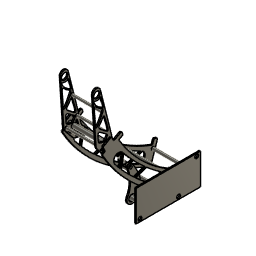
Klapptriebwerk v25 (Autodesk Fusion 360 design; units mm, degrees)
Autodesk Fusion 360 part; units mm, degrees
note: some values were not read from the file. Set by a fixed rule: which face or edge a step refers to.
(part 1 of 2)
sketch "Sketch2" plane through (0, 0, 0) normal (1, 0, 0) x (0, 1, 0)
  line L0 (125, -60) -> (-125, -60)
  line L1 (-125, -60) -> (-125, 60)
  line L2 (-125, 60) -> (125, 60)
  line L3 (125, 60) -> (125, -60)
  line L4 (125, -60) -> (-125, 60) construction
  line L5 (-125, -60) -> (125, 60) construction
  arc A0 (-186.1426, 249.5286) -> (95.8875, 14.6255) centre (286.6925, 530.468) ccw
  arc A1 (-250.577, 231.1913) -> (89.5042, -52.0625) centre (286.6925, 530.468) ccw
  line L6 (112.4731, 8.7903) -> (92.6771, -50.4864)
  line L7 (-240.9623, 242.2177) -> (-248.2082, 255.3516)
  line L8 (-247.2269, 258.7482) -> (-218.7703, 274.4476)
  line L9 (-215.3737, 273.4663) -> (-208.1278, 260.3325)
  line L10 (-223.3374, 249.0861) -> (-254.8183, 306.148) construction
  line L11 (-194.8808, 264.7856) -> (-204.7312, 259.3511)
  line L12 (-241.9437, 238.8211) -> (-249.6006, 234.5968)
  line L13 (-194.8808, 264.7856) -> (-179.3789, 273.3379)
  line L14 (-175.9823, 272.3566) -> (-171.1517, 263.6007)
  line L15 (-172.133, 260.2041) -> (-185.201, 252.9945)
  line L16 (112.4731, 8.7903) -> (118.0165, 25.3892)
  line L17 (116.4371, 28.5523) -> (106.9521, 31.72)
  line L18 (103.7889, 30.1406) -> (99.1261, 16.1784)
  arc A2 (-185.201, 252.9945) -> (-186.1426, 249.5286) centre (-183.9934, 250.8056) ccw
  arc A3 (-172.133, 260.2041) -> (-171.1517, 263.6007) centre (-173.3407, 262.3931) ccw
  arc A4 (-175.9823, 272.3566) -> (-179.3789, 273.3379) centre (-178.1713, 271.1489) ccw
  arc A5 (-208.1278, 260.3325) -> (-204.7312, 259.3511) centre (-205.9388, 261.5401) ccw
  arc A6 (-215.3737, 273.4663) -> (-218.7703, 274.4476) centre (-217.5627, 272.2586) ccw
  arc A7 (-247.2269, 258.7482) -> (-248.2082, 255.3516) centre (-246.0193, 256.5592) ccw
  arc A8 (-241.9437, 238.8211) -> (-240.9623, 242.2177) centre (-243.1513, 241.0101) ccw
  arc A9 (-249.6006, 234.5968) -> (-250.577, 231.1913) centre (-248.3929, 232.4079) ccw
  arc A10 (89.5042, -52.0625) -> (92.6771, -50.4864) centre (90.3058, -49.6945) ccw
  arc A11 (118.0165, 25.3892) -> (116.4371, 28.5523) centre (115.6452, 26.1811) ccw
  arc A12 (106.9521, 31.72) -> (103.7889, 30.1406) centre (106.1602, 29.3487) ccw
  arc A13 (95.8875, 14.6255) -> (99.1261, 16.1784) centre (96.7548, 16.9703) ccw
  arc A14 (8.8006, 55.8354) -> (95.8875, 14.6255) centre (286.6925, 530.468) ccw
  arc A15 (10.0637, 57.9928) -> (96.7548, 16.9703) centre (286.6925, 530.468) ccw
  line L19 (96.7548, 16.9703) -> (95.8875, 14.6255)
  line L20 (10.0637, 57.9928) -> (8.8006, 55.8354)
  arc A16 (-94.5095, 47.8604) -> (89.5042, -52.0625) centre (286.6925, 530.468) ccw
  arc A17 (-96.0591, 45.8986) -> (88.7027, -54.4305) centre (286.6925, 530.468) ccw
  line L21 (88.7027, -54.4305) -> (89.5042, -52.0625)
  line L22 (-96.0591, 45.8986) -> (-94.5095, 47.8604)
  line L23 (324.1005, 496.8726) -> (249.2844, 496.8726)
  line L24 (249.2844, 496.8726) -> (249.2844, 564.0634)
  line L25 (249.2844, 564.0634) -> (324.1005, 564.0634)
  line L26 (324.1005, 564.0634) -> (324.1005, 496.8726)
  line L27 (324.1005, 496.8726) -> (249.2844, 564.0634) construction
  line L28 (249.2844, 496.8726) -> (324.1005, 564.0634) construction
  circle A18 centre (-223.3374, 249.0861) radius 15
  circle A19 centre (-223.3374, 249.0861) radius 8.5
  point P0 (-249.4159, 257.5405)
  point P1 (-216.5813, 275.6552)
  point P2 (-206.9201, 258.1435)
  point P3 (-177.1899, 274.5456)
  point P4 (-169.944, 261.4117)
  point P5 (-187.4558, 251.7506)
  point P6 (118.8084, 27.7604)
  point P7 (104.5808, 32.5119)
  point P8 (286.6925, 530.468)
  point P9 (286.6925, 530.468)
  dimension "d1" = 250
  dimension "d2" = 120
  dimension "d12" = 20
  dimension "d13" = 400
  dimension "d14" = 550
  dimension "d17" = 37.5
  dimension "d18" = 13.75
  dimension "d19" = 20
  dimension "d20" = 15
  dimension "d22" = 15
  dimension "d23" = 20
  dimension "d24" = 2.5
  dimension "d25" = -2.5
  dimension "d26" = 2.5
  dimension "d44" = 30
  dimension "d45" = 17
  constraint horizontal L0
  constraint perpendicular L0 L1
  constraint parallel L0 L2
  constraint parallel L1 L3
  constraint coincident L4 origin
  constraint coincident L5 origin
  constraint perpendicular L7 L8
  constraint perpendicular L9 L11
  constraint perpendicular L10 L11
  constraint perpendicular L7 L11
  constraint symmetric L7 L9 L10
  constraint collinear L11 L12
  constraint coincident L10.start L11
  constraint parallel L11 L13
  constraint perpendicular L13 L14
  constraint coincident A0 P5
  constraint perpendicular L14 L15
  constraint parallel L6 L16
  constraint perpendicular L16 L17
  constraint perpendicular L17 L18
  constraint concentric A0 A1
  constraint tangent L15 A2
  constraint tangent A0 A2
  constraint coincident P4 L14
  constraint coincident P4 L15
  constraint tangent L14 A3
  constraint tangent L15 A3
  constraint equal A2 A3
  constraint coincident P3 L13
  constraint coincident P3 L14
  constraint tangent L13 A4
  constraint tangent L14 A4
  constraint equal A2 A4
  constraint coincident P2 L9
  constraint coincident P2 L11
  constraint tangent L9 A5
  constraint tangent L11 A5
  constraint equal A2 A5
  constraint coincident P1 L8
  constraint coincident P1 L9
  constraint tangent L8 A6
  constraint tangent L9 A6
  constraint equal A2 A6
  constraint coincident P0 L7
  constraint coincident P0 L8
  constraint tangent L7 A7
  constraint tangent L8 A7
  constraint equal A2 A7
  constraint tangent L7 A8
  constraint tangent L12 A8
  constraint equal A2 A8
  constraint tangent A1 A9
  constraint tangent L12 A9
  constraint equal A2 A9
  constraint tangent A1 A10
  constraint tangent L6 A10
  constraint equal A2 A10
  constraint coincident P6 L16
  constraint coincident P6 L17
  constraint tangent L16 A11
  constraint tangent L17 A11
  constraint equal A2 A11
  constraint coincident P7 L17
  constraint coincident P7 L18
  constraint tangent L17 A12
  constraint tangent L18 A12
  constraint equal A2 A12
  constraint tangent L18 A13
  constraint tangent A0 A13
  constraint equal A2 A13
  constraint coincident A0 A14.start
  constraint tangent A13 A14
  constraint coincident A13.centre A15.end
  constraint coincident A1 A16.start
  constraint coincident P9 P8
  constraint horizontal L23
  constraint perpendicular L23 L24
  constraint parallel L23 L25
  constraint parallel L24 L26
  constraint coincident L27 P9
  constraint coincident L28 P9
  constraint coincident P8 A0.centre
  constraint coincident L10.start A18.centre
  constraint concentric A18 A19
  measures "d1" distance of L1.end L2.end
  measures "d2" distance of L0.end L1.end
  measures "d12" distance of P1 P2
  measures "d13" distance of L11.start L6.start
  measures "d14" radius of A0
  measures "d17" distance of P0 P1
  measures "d18" distance of L11.start P2
  measures "d19" distance of L6.start P6
  measures "d20" distance of P6 P7
  measures "d22" distance of P3 P4
  measures "d23" distance of P4 P5
  measures "d24" radius of A2
  measures "d44" diameter of A18
  measures "d45" diameter of A19
extrude "Extrude1" add sketch "Sketch2" along normal blind 5 contours L0 L1 L2 L3 A0 A1 L6 L16 L17 L18 A10 A11 A12 A13 A15 L19 L20 A17 L21 L22 | L2 A0 A1 L6 L16 L17 L18 A10 A11 A12 A13 A14 A16 | A0 A14 A15 L19 L20 | A1 A16 A17 L21 L22 makes body 1
extrude "Extrude2" add sketch "Sketch2" against normal blind 5 contours A0 A14 A15 L19 L20 | A1 A16 A17 L21 L22 bodies 1
extrude "Extrude3" add sketch "Sketch2" against normal blind 5 separate body contours L2 A0 A1 L6 L16 L17 L18 A10 A11 A12 A13 A14 A16 | L2 A0 A1 L7 L8 L9 L11 L12 L13 L14 L15 A2 A3 A4 A5 A6 A7 A8 A9 | A18 | A19 makes body 2
extrude "Extrude4" add sketch "Sketch2" along normal blind 1 separate body contours L23 L24 L25 L26 makes body 3
copy_body "Body->Comp1" bodies 2 removing the originals makes body 4 in component "Brazo_inferior"
copy_body "Body->Comp2" bodies 1 removing the originals makes body 5 in component "Base"
extrude "Extrude1'" add sketch "Sketch2" against normal blind 80 from surface at -5 contours A19 bodies 4 in component "Brazo_inferior"
ref_plane "WorkPlane1" through (-15, -66.137, 111.6299) normal (-1, 0, 0) x (0, -1, 0)
sketch "Sketch5" plane through (-15, 0, 0) normal (-1, 0, 0) x (0, -1, 0)
  circle A0 centre (223.3374, 249.0861) radius 8.5
  line L0 (178.7602, 194.3477) -> (215.6605, 202.9742)
  line L1 (226.6871, 209.9081) -> (256.5218, 246.971)
  line L2 (260.8937, 258.1191) -> (273.342, 436.4099)
  line L3 (243.8201, 441.0681) -> (194.2709, 241.4386)
  line L4 (189.4633, 232.5912) -> (169.1821, 210.9178)
  arc A1 (273.342, 436.4099) -> (243.8201, 441.0681) centre (258.3784, 437.4547) ccw
  arc A2 (169.1821, 210.9178) -> (178.7602, 194.3477) centre (176.4838, 204.0852) ccw
  circle A3 centre (176.4838, 204.0852) radius 5
  arc A4 (189.4633, 232.5912) -> (194.2709, 241.4386) centre (174.8599, 246.2565) ccw
  arc A5 (215.6605, 202.9742) -> (226.6871, 209.9081) centre (211.1076, 222.4491) ccw
  arc A6 (256.5218, 246.971) -> (260.8937, 258.1191) centre (240.9423, 259.5121) ccw
  point P0 (260.4567, 251.8592)
  dimension "d58" = 20
  dimension "d60" = 185
  dimension "d61" = 10
  dimension "d62" = 20
  dimension "d63" = 15
  constraint tangent L0 A2
  constraint tangent L4 A2
  constraint tangent L2 A1
  constraint concentric A2 A3
  constraint tangent L3 A4
  constraint tangent L4 A4
  constraint tangent L0 A5
  constraint tangent L1 A5
  constraint equal A4 A5
  constraint coincident P0 L1
  constraint coincident P0 L2
  constraint tangent L1 A6
  constraint tangent L2 A6
  constraint equal A4 A6
  constraint tangent L3 A1
  measures "d58" diameter of A2
  measures "d60" distance of P0 L2.end
  measures "d61" diameter of A3
  measures "d62" radius of A4
  measures "d63" radius of A1
extrude "Extrude5" add sketch "Sketch5" along normal blind 5 separate body makes body 6
copy_body "Body->Comp3" bodies 6 removing the originals makes body 7 in component "Brazo_superior"
extrude "Extrude6" add sketch "Sketch5" along normal blind 50 from surface at 5 separate body contours A3 makes body 8
combine "Combine1" operation add target body 7 tool bodies 8 in component "Brazo_superior"
ref_plane "WorkPlane2" through (-45, -219.207, 323.537) normal (-1, 0, 0) x (0, -1, 0)
sketch "Sketch6" plane through (-45, 0, 0) normal (-1, 0, 0) x (0, -1, 0)
  circle A0 centre (176.4838, 204.0852) radius 5
  line L0 (176.4838, 204.0852) -> (212.8748, 179.6652) construction
  line L1 (176.4838, 204.0852) -> (219.4836, 212.55) construction
  line L2 (176.4838, 204.0852) -> (152.8065, 168.8009) construction
  line L3 (181.8086, 198.8034) -> (173.0057, 189.9288)
  line L4 (169.5779, 207.0107) -> (164.702, 195.5009)
  line L5 (164.702, 195.5009) -> (173.0057, 189.9288)
  line L6 (170.0994, 191.8791) -> (145.0247, 154.5125)
  line L7 (145.0247, 154.5125) -> (147.1006, 153.1194)
  line L8 (147.1006, 153.1194) -> (146.5434, 152.2891)
  line L9 (146.5434, 152.2891) -> (144.4675, 153.6821)
  line L10 (173.1539, 214.2939) -> (194.1567, 203.2991) construction
  line L11 (145.7207, 155.3702) -> (148.627, 153.4199)
  line L12 (148.627, 153.4199) -> (121.825, 113.4792)
  line L13 (121.825, 113.4792) -> (118.9187, 115.4294)
  line L14 (145.1635, 154.5398) -> (147.2394, 153.1467)
  line L15 (147.2394, 153.1467) -> (121.5518, 114.8668)
  line L16 (121.5518, 114.8668) -> (119.4759, 116.2598)
  line L17 (145.1635, 154.5398) -> (145.7207, 155.3702)
  line L18 (119.4759, 116.2598) -> (118.9187, 115.4294)
  line L19 (144.4675, 153.6821) -> (143.222, 154.5179)
  line L20 (143.222, 154.5179) -> (168.8538, 192.7149)
  line L21 (145.5055, 152.9856) -> (146.6756, 154.7294) construction
  line L22 (146.0905, 153.8575) -> (155.0061, 147.8747) construction
  line L23 (146.822, 152.7042) -> (154.8831, 147.2949) construction
  arc A1 (181.8086, 198.8034) -> (169.5779, 207.0107) centre (176.4838, 204.0852) ccw
  line L24 (117.6458, 116.404) -> (105.3249, 98.0433) construction
  circle A2 centre (109.9601, 104.9507) radius 5
  line L25 (113.4383, 119.107) -> (121.7419, 113.5349)
  line L26 (104.6353, 110.2324) -> (113.4383, 119.107)
  arc A3 (104.6353, 110.2324) -> (116.866, 102.0251) centre (109.9601, 104.9507) ccw
  line L27 (116.866, 102.0251) -> (121.7419, 113.5349)
  dimension "d69" = 15
  dimension "d70" = 45
  dimension "d71" = 5
  dimension "d77" = 45
  dimension "d78" = 1.5
  dimension "d79" = 2.5
  dimension "d80" = 1
  dimension "d81" = 2.5
  dimension "d83" = 1
  dimension "d85" = 0.1
  dimension "d86" = 0.1
  dimension "d87" = 0.1
  dimension "d88" = 3.5
  dimension "d89" = 12.5
  dimension "d90" = 1.6
  dimension "d91" = 10
  constraint concentric A0 A1
  constraint coincident A0.centre L0.start
  constraint perpendicular L0 L2
  constraint tangent L3 A1
  constraint symmetric L2 L3.end L4.end
  constraint coincident L5 L6.start
  constraint perpendicular L6 L7
  constraint perpendicular L7 L8
  constraint perpendicular L8 L9
  constraint parallel L2 L6
  constraint tangent L10 A1
  constraint perpendicular L11 L12
  constraint perpendicular L12 L13
  constraint perpendicular L11 L17
  constraint perpendicular L13 L18
  constraint parallel L6 L17
  constraint perpendicular L2 L19
  constraint midpoint L5 L20.end
  constraint perpendicular L5 L20
  constraint midpoint L9 L21.start
  constraint coincident L11 L21.end
  constraint perpendicular L11 L21
  constraint midpoint L21 L22.start
  constraint perpendicular L21 L22
  constraint midpoint L8 L23.start
  constraint perpendicular L8 L23
  constraint tangent L4 A1
  constraint symmetric L3.end L19 L25.end
  constraint symmetric L4.end L19 L25.start
  constraint symmetric L19 L4.start L26.start
  constraint symmetric L19 L3.start A3.end
  constraint symmetric L19 A1 A3
  constraint coincident A2.centre A3.centre
  constraint collinear L13 L25
  measures "d69" diameter of A1
  measures "d70" angle of L0 L1
  measures "d71" distance of L2 L3.end
  measures "d77" distance of L6.start L6.end
  measures "d78" distance of L2 L6
  measures "d79" distance of L6.end L7.end
  measures "d80" distance of L7.end L8.end
  measures "d81" distance of L8.end L9.end
  measures "d85" distance of L6 L17
  measures "d86" distance of L8 L15
  measures "d87" distance of L7 L14
  measures "d88" distance of L12.end L13.end
  measures "d89" distance of L3.end L3.start
  measures "d90" distance of L18 L24
  measures "d91" diameter of A2
extrude "Extrude7" add sketch "Sketch6" along normal blind 5 separate body contours L3 L4 L5 A1 makes body 9
ref_plane "WorkPlane3" through (-47.5, -175.0122, 200.7669) normal (-1, 0, 0) x (0, -1, 0)
sketch "Sketch7" plane through (-47.5, 0, 0) normal (-1, 0, 0) x (0, -1, 0)
  line L0 (143.222, 154.5179) -> (168.8538, 192.7149)
  line L1 (145.0247, 154.5125) -> (147.1006, 153.1194)
  line L2 (147.1006, 153.1194) -> (146.5434, 152.2891)
  line L3 (146.5434, 152.2891) -> (144.4675, 153.6821)
  line L4 (144.4675, 153.6821) -> (143.222, 154.5179)
  line L5 (143.222, 154.5179) -> (168.8538, 192.7149)
  line L6 (170.0994, 191.8791) -> (145.0247, 154.5125)
  line L7 (119.4759, 116.2598) -> (118.9187, 115.4294)
  line L8 (121.5518, 114.8668) -> (119.4759, 116.2598)
  line L9 (147.2394, 153.1467) -> (121.5518, 114.8668)
  line L10 (145.1635, 154.5398) -> (147.2394, 153.1467)
  line L11 (145.1635, 154.5398) -> (145.7207, 155.3702)
  line L12 (145.7207, 155.3702) -> (148.627, 153.4199)
  line L13 (121.825, 113.4792) -> (118.9187, 115.4294)
  line L14 (148.627, 153.4199) -> (121.825, 113.4792)
  line L15 (170.0994, 191.8791) -> (168.8538, 192.7149)
  constraint coincident L6.start L15.start
  constraint coincident L0.end L5.end
revolve "Revolve1" add sketch "Sketch7" angle 360 about axis through (-47.5, -143.222, 154.5179) along (0, -0.557214, 0.830369) contours L0 L1 L2 L3 L4 L5 L6 L15 bodies 9
revolve "Revolve2" add sketch "Sketch7" angle 360 about axis through (-47.5, -143.222, 154.5179) along (0, -0.557214, 0.830369) separate body contours L7 L8 L9 L10 L11 L12 L13 L14 makes body 10
extrude "Extrude8" add sketch "Sketch6" along normal blind 8 and the other way blind 3 contours L13 L25 L26 A3 L27 bodies 10
extrude "Extrude9" add sketch "Sketch6" along normal blind 10 and the other way blind 15 separate body contours A2 makes body 11
ref_plane "WorkPlane4" through (-36, -111.4317, 108.2689) normal (1, 0, 0) x (0, 1, 0)
sketch "Sketch8" plane through (-36, 0, 0) normal (1, 0, 0) x (0, 1, 0)
  circle A0 centre (-109.9601, 104.9507) radius 5
  line L0 (0, 0) -> (-206.999, 0) construction
  line L1 (-122.3205, 10) -> (-101.7641, 45.6047) construction
  line L2 (-101.7641, 45.6047) -> (-119.4988, 101.9483) construction
  spline S0 degree 2 poles (-122.3205, 10) (-101.7641, 45.6047) (-119.4988, 101.9483) knots 0 0 0 1 1 1
  line L3 (-91.6181, -14.8636) -> (-46.7056, 25.5718) construction
  line L4 (-46.7056, 25.5718) -> (-101.5636, 110.3819) construction
  spline S1 degree 2 poles (-91.6181, -14.8636) (-46.7056, 25.5718) (-101.5636, 110.3819) knots 0 0 0 1 1 1
  line L5 (-125, -60) -> (-125, 60)
  circle A1 centre (-105, 0) radius 12.5
  arc A2 (-101.5636, 110.3819) -> (-119.4988, 101.9483) centre (-109.9601, 104.9507) ccw
  arc A3 (-122.3205, 10) -> (-91.6181, -14.8636) centre (-105, 0) ccw
  circle A4 centre (-105, 0) radius 7.5
  dimension "d107" = 20
  dimension "d108" = 40
  dimension "d109" = 20
  dimension "d110" = 25
  dimension "d113" = 15
  constraint concentric A0 A2
  constraint coincident L0.start origin
  constraint horizontal L0
  constraint coincident A1.centre L0
  constraint tangent S0 A3
  constraint tangent S1 A3
  constraint tangent S1 A2
  constraint tangent S0 A2
  constraint concentric A1 A3
  constraint concentric A1 A4
  measures "d107" diameter of A2
  measures "d108" diameter of A3
  measures "d109" distance of A1.centre L5
  measures "d110" diameter of A1
  measures "d113" diameter of A4
extrude "Extrude10" add sketch "Sketch8" along normal blind 5 separate body contours S0 S1 A2 A3 makes body 12
extrude "Extrude1''" add sketch "Sketch8" along normal up to surface (36 mm away) contours A4 bodies 5 in component "Base"
copy_body "Body->Comp4" bodies 11 removing the originals makes body 13 in component "Axis_slider_crank"
copy_body "Body->Comp5" bodies 9 removing the originals makes body 14 in component "SliderUp"
copy_body "Body->Comp6" bodies 10 removing the originals makes body 15 in component "SliderBot"
copy_body "Body->Comp7" bodies 12 removing the originals makes body 16 in component "Crank"
sketch "Sketch1" plane through (0, 0, 0) normal (-1, 0, 0) x (0, -1, 0) in component "Base"
  circle A0 centre (105, 0) radius 7.5
  arc A1 (-89.5042, -52.0625) -> (94.5095, 47.8604) centre (-286.6925, 530.468) ccw
  line L0 (94.5095, 47.8604) -> (96.0591, 45.8986)
  arc A2 (-88.7027, -54.4305) -> (96.0591, 45.8986) centre (-286.6925, 530.468) ccw
  line L1 (-88.7027, -54.4305) -> (-89.5042, -52.0625)
  line L2 (-10.0637, 57.9928) -> (-8.8006, 55.8354)
  arc A3 (-95.8875, 14.6255) -> (-8.8006, 55.8354) centre (-286.6925, 530.468) ccw
  line L3 (-95.8875, 14.6255) -> (-96.7548, 16.9703)
  arc A4 (-96.7548, 16.9703) -> (-10.0637, 57.9928) centre (-286.6925, 530.468) ccw
  line L4 (125, 60) -> (-125, 60)
  line L5 (-125, 60) -> (-125, -60)
  line L6 (-125, -60) -> (125, -60)
  line L7 (125, -60) -> (125, 60)
  circle A5 centre (-40, -50) radius 7.5
  circle A6 centre (-110, 50) radius 7.5
  circle A7 centre (110, -50) radius 7.5
  dimension "d177" = 15
  dimension "d178" = 15
  dimension "d179" = 15
  dimension "d180" = 10
  dimension "d181" = 10
  dimension "d182" = 15
  dimension "d183" = 40
  dimension "d184" = 15
  dimension "d185" = 10
  measures "d177" diameter of A5
  measures "d178" diameter of A6
  measures "d179" diameter of A7
  measures "d180" distance of L6 A7.centre
  measures "d181" distance of L6 A5.centre
  measures "d182" distance of L7 A7.centre
  measures "d183" horizontal distance of origin A5.centre
  measures "d184" distance of L5 A6.centre
  measures "d185" distance of L4 A6.centre
extrude "Extrude2'" cut sketch "Sketch1" against normal through all contours A5 | A6 | A7 bodies 5 in component "Base"
other "Base Mesh Feature1"
sketch "Sketch12" plane through (0, 0, 0) normal (1, 0, 0) x (0, 1, 0)
  line L0 (-241.9437, 238.8211) -> (-249.6006, 234.5968)
  arc A0 (-249.6006, 234.5968) -> (-250.577, 231.1913) centre (-248.3929, 232.4079) ccw
  arc A1 (-250.577, 231.1913) -> (89.5042, -52.0625) centre (286.6925, 530.468) ccw
  arc A2 (89.5042, -52.0625) -> (92.6771, -50.4864) centre (90.3058, -49.6945) ccw
  line L1 (92.6771, -50.4864) -> (118.0165, 25.3892)
  arc A3 (118.0165, 25.3892) -> (116.4371, 28.5523) centre (115.6452, 26.1811) ccw
  line L2 (116.4371, 28.5523) -> (106.9521, 31.72)
  arc A4 (106.9521, 31.72) -> (103.7889, 30.1406) centre (106.1602, 29.3487) ccw
  line L3 (103.7889, 30.1406) -> (99.1261, 16.1784)
  arc A5 (95.8875, 14.6255) -> (99.1261, 16.1784) centre (96.7548, 16.9703) ccw
  arc A6 (-186.1426, 249.5286) -> (95.8875, 14.6255) centre (286.6925, 530.468) ccw
  arc A7 (-185.201, 252.9945) -> (-186.1426, 249.5286) centre (-183.9934, 250.8056) ccw
  line L4 (-185.201, 252.9945) -> (-172.133, 260.2041)
  arc A8 (-172.133, 260.2041) -> (-171.1517, 263.6007) centre (-173.3407, 262.3931) ccw
  line L5 (-171.1517, 263.6007) -> (-175.9823, 272.3566)
  arc A9 (-175.9823, 272.3566) -> (-179.3789, 273.3379) centre (-178.1713, 271.1489) ccw
  line L6 (-179.3789, 273.3379) -> (-204.7312, 259.3511)
  arc A10 (-208.1278, 260.3325) -> (-204.7312, 259.3511) centre (-205.9388, 261.5401) ccw
  line L7 (-208.1278, 260.3325) -> (-215.3737, 273.4663)
  arc A11 (-215.3737, 273.4663) -> (-218.7703, 274.4476) centre (-217.5627, 272.2586) ccw
  line L8 (-218.7703, 274.4476) -> (-247.2269, 258.7482)
  arc A12 (-247.2269, 258.7482) -> (-248.2082, 255.3516) centre (-246.0193, 256.5592) ccw
  line L9 (-248.2082, 255.3516) -> (-240.9623, 242.2177)
  arc A13 (-241.9437, 238.8211) -> (-240.9623, 242.2177) centre (-243.1513, 241.0101) ccw
  arc A14 (-172.3826, 202.0689) -> (59.1497, 12.5724) centre (380.3227, 641.1856) ccw
  arc A15 (-172.3826, 202.0689) -> (-203.1179, 177.6501) centre (-187.7502, 189.8595) ccw
  arc A16 (-203.1179, 177.6501) -> (41.2897, -22.384) centre (380.3227, 641.1856) ccw
  arc A17 (41.2897, -22.384) -> (59.1497, 12.5724) centre (50.2197, -4.9058) ccw
  arc A18 (-187.7502, 189.8595) -> (50.2197, -4.9058) centre (380.3227, 641.1856) ccw construction
  line L10 (-172.3826, 202.0689) -> (-181.3078, 151.4518)
  line L11 (-168.2204, 196.8803) -> (-177.0785, 146.6434)
  line L12 (-126.061, 94.5198) -> (-84.2819, 109.7261)
  line L13 (-121.9147, 90.708) -> (-79.9597, 105.9784)
  line L14 (-23.7809, 62.3878) -> (-31.2551, 19.9998)
  line L15 (-19.2562, 59.2549) -> (-26.7053, 17.0091)
  line L16 (59.8059, 12.2376) -> (10.4773, -5.7166)
  line L17 (53.7571, 15.3569) -> (4.8259, -2.4526)
  line L18 (-187.7502, 189.8595) -> (-107.7603, 189.8595) construction
  arc A19 (95.8875, 14.6255) -> (112.442, 8.697) centre (389.3923, 808.1176) ccw construction
  arc A20 (-186.1426, 249.5286) -> (-195.2632, 264.5746) centre (-1041.8296, -258.886) ccw construction
  line L19 (112.442, 8.697) -> (92.6771, -50.4864) construction
  line L20 (-195.2632, 264.5746) -> (-249.6006, 234.5968) construction
  arc A21 (-222.4319, 249.5857) -> (102.5595, -20.8947) centre (294.6052, 540.3391) ccw construction
  dimension "d238" = 5
  dimension "d239" = 5
  dimension "d240" = 5
  dimension "d241" = 5
  dimension "d242" = 100
  dimension "d246" = 60
  dimension "d247" = 60
  dimension "d248" = 60
  dimension "d249" = 145
  dimension "d250" = 132.3537
  constraint tangent A14 A15
  constraint tangent A15 A16
  constraint tangent A16 A17
  constraint tangent A14 A17
  constraint coincident A16 L10.end
  constraint coincident A14 L11.start
  constraint coincident A16 L11.end
  constraint parallel L10 L11
  constraint coincident A16 L12.start
  constraint coincident A14 L12.end
  constraint coincident A16 L13.start
  constraint coincident A14 L13.end
  constraint parallel L12 L13
  constraint coincident A14 L14.start
  constraint coincident A16 L14.end
  constraint coincident A14 L15.start
  constraint coincident A16 L15.end
  constraint parallel L14 L15
  constraint coincident A14 L16.start
  constraint coincident A16 L16.end
  constraint coincident A14 L17.start
  constraint coincident A16 L17.end
  constraint parallel L16 L17
  constraint coincident A15.centre A18.start
  constraint horizontal L18
  constraint tangent A5 A19
  constraint coincident L1 A19.end
  constraint coincident A5.start A6.end
  constraint tangent A7 A20
  constraint coincident L6 A20.end
  constraint coincident A6.start A7.end
  constraint coincident A2.end L1.start
  constraint coincident L0.end A0.start
  constraint tangent A18 A21
  constraint midpoint L19 A21.end
  constraint midpoint L20 A21.start
  measures "d238" distance of L10 L11
  measures "d239" distance of L12 L13
  measures "d240" distance of L14 L15
  measures "d241" distance of L16 L17
  measures "d242" angle of L10 L18
  measures "d246" angle of L11 L12
  measures "d247" angle of L13 L14
  measures "d248" angle of L15 L17
  measures "d249" distance of A1.centre A14.centre
  measures "d250" distance of A14.centre A21.centre
extrude "Extrude4'" cut sketch "Sketch12" against normal through all contours A15 A16 L10 | A14 A16 L11 L12 | A14 A16 L13 L14 | A14 A16 L15 L17 | A16 A17 L16 bodies 4 in component "Brazo_inferior"
other "Base Mesh Feature2"
sketch "Sketch13" plane through (-15, 0, 0) normal (1, 0, 0) x (0, 1, 0)
  circle A0 centre (-223.3374, 249.0861) radius 8.5
  circle A1 centre (-176.4838, 204.0852) radius 5
  line L0 (-169.1821, 210.9178) -> (-189.4633, 232.5912)
  arc A2 (-194.2709, 241.4386) -> (-189.4633, 232.5912) centre (-174.8599, 246.2565) ccw
  line L1 (-194.2709, 241.4386) -> (-243.8201, 441.0681)
  arc A3 (-243.8201, 441.0681) -> (-273.342, 436.4099) centre (-258.3784, 437.4547) ccw
  line L2 (-273.342, 436.4099) -> (-260.8937, 258.1191)
  arc A4 (-260.8937, 258.1191) -> (-256.5218, 246.971) centre (-240.9423, 259.5121) ccw
  line L3 (-256.5218, 246.971) -> (-226.6871, 209.9081)
  arc A5 (-226.6871, 209.9081) -> (-215.6605, 202.9742) centre (-211.1076, 222.4491) ccw
  line L4 (-215.6605, 202.9742) -> (-178.7602, 194.3477)
  arc A6 (-178.7602, 194.3477) -> (-169.1821, 210.9178) centre (-176.4838, 204.0852) ccw
  spline S0 degree 3 poles (-243.6188, 239.3572) (-227.1439, 245.9013) (-225.7976, 239.2027) (-231.4249, 227.1643) knots 0.175444 0.175444 0.175444 0.175444 0.949588 0.949588 0.949588 0.949588
  line L5 (-243.9542, 237.7182) -> (-233.0354, 226.8781)
  arc A7 (-243.6188, 239.3572) -> (-243.9542, 237.7182) centre (-243.2497, 238.4278) ccw
  arc A8 (-233.0354, 226.8781) -> (-231.4249, 227.1643) centre (-232.3308, 227.5878) ccw
  line L6 (-243.6188, 239.3572) -> (-227.1439, 245.9013) construction
  line L7 (-227.1439, 245.9013) -> (-225.7976, 239.2027) construction
  line L8 (-225.7976, 239.2027) -> (-231.4249, 227.1643) construction
  line L9 (-211.9586, 262.8712) -> (-213.9, 262.5) construction
  line L10 (-213.9, 262.5) -> (-215, 260) construction
  line L11 (-215, 260) -> (-215, 257) construction
  line L12 (-215, 257) -> (-212.5679, 252.5298) construction
  line L13 (-212.5679, 252.5298) -> (-212.2678, 249.9329) construction
  line L14 (-212.2678, 249.9329) -> (-212.5261, 247.5635) construction
  line L15 (-212.5261, 247.5635) -> (-214.6128, 241.6791) construction
  line L16 (-214.6128, 241.6791) -> (-217, 240) construction
  line L17 (-217, 240) -> (-218.5775, 235.2522) construction
  line L18 (-218.5775, 235.2522) -> (-220, 231) construction
  line L19 (-220, 231) -> (-221, 229) construction
  line L20 (-221, 229) -> (-220.5807, 226.196) construction
  line L21 (-220.5807, 226.196) -> (-217.5759, 223.692) construction
  line L22 (-217.5759, 223.692) -> (-213.5278, 221.7305) construction
  line L23 (-213.5278, 221.7305) -> (-209.5631, 220.0194) construction
  line L24 (-209.5631, 220.0194) -> (-204.555, 219.2265) construction
  line L25 (-204.555, 219.2265) -> (-203, 220) construction
  line L26 (-203, 220) -> (-201.592, 223.2329) construction
  line L27 (-201.592, 223.2329) -> (-202, 228) construction
  line L28 (-202, 228) -> (-201.9676, 233.4159) construction
  line L29 (-201.9676, 233.4159) -> (-203.5534, 240.5523) construction
  line L30 (-203.5534, 240.5523) -> (-204.8472, 246.5619) construction
  line L31 (-204.8472, 246.5619) -> (-206.5583, 254.533) construction
  line L32 (-206.5583, 254.533) -> (-209.5, 263.2) construction
  line L33 (-209.5, 263.2) -> (-210.4715, 262.8927) construction
  line L34 (-210.4715, 262.8927) -> (-211.9586, 262.8712) construction
  spline S1 degree 5 poles (-211.9586, 262.8712) (-213.9, 262.5) (-215, 260) (-215, 257) (-212.5679, 252.5298) (-212.2678, 249.9329) (-212.5261, 247.5635) (-214.6128, 241.6791) (-217, 240) (-218.5775, 235.2522) (-220, 231) (-221, 229) (-220.5807, 226.196) (-217.5759, 223.692) (-213.5278, 221.7305) (-209.5631, 220.0194) (-204.555, 219.2265) (-203, 220) (-201.592, 223.2329) (-202, 228) (-201.9676, 233.4159) (-203.5534, 240.5523) (-204.8472, 246.5619) (-206.5583, 254.533) (-209.5, 263.2) (-210.4715, 262.8927) (-211.9586, 262.8712) knots 0 0 0 0 0 0 0.045455 0.090909 0.136364 0.181818 0.227273 0.272727 0.318182 0.363636 0.409091 0.454545 0.5 0.545455 0.590909 0.636364 0.681818 0.727273 0.772727 0.818182 0.863636 0.909091 0.954545 1 1 1 1 1 1
  spline S2 degree 5 poles (-227.3096, 258.9797) (-226.9432, 259.1978) (-226.2016, 259.7451) (-225.0348, 260.8843) (-223.2769, 262.8723) (-220.9461, 265.8348) (-218.8092, 268.9034) (-217.2191, 271.7616) (-216.4409, 274.1709) (-216.3575, 275.9607) (-216.9709, 277.3411) (-218.3999, 278.723) (-220.7214, 280.4961) (-223.8779, 282.8245) (-227.7009, 285.6855) (-231.9484, 288.9151) (-236.3362, 292.2511) (-240.5719, 295.3758) (-244.387, 297.9591) (-247.5704, 299.7014) (-250.0012, 300.3759) (-251.6838, 299.8733) (-252.7099, 298.1966) (-253.2192, 295.4532) (-253.3561, 291.8523) (-253.2502, 287.6795) (-253.0108, 283.2567) (-252.7167, 278.9076) (-252.4087, 274.921) (-252.0792, 271.5133) (-251.6662, 268.796) (-251.0366, 266.7268) (-250.0265, 265.154) (-248.5043, 263.8975) (-246.4235, 262.8169) (-243.8891, 261.8877) (-241.1096, 261.1639) (-238.3081, 260.6365) (-235.6845, 260.2815) (-233.2736, 259.6803) (-231.0644, 258.7491) (-229.4862, 258.2952) (-228.3997, 258.4361) (-227.6759, 258.7615) (-227.3096, 258.9797) knots 0 0 0 0 0 0 0.025 0.05 0.075 0.1 0.125 0.15 0.175 0.2 0.225 0.25 0.275 0.3 0.325 0.35 0.375 0.4 0.425 0.45 0.475 0.5 0.525 0.55 0.575 0.6 0.625 0.65 0.675 0.7 0.725 0.75 0.775 0.8 0.825 0.85 0.875 0.9 0.925 0.95 0.975 1 1 1 1 1 1
  line L35 (-244.2372, 261.9439) -> (-227.0166, 258.4573)
  line L36 (-231.9908, 256.1921) -> (-222.6284, 261.7673)
  line L37 (-218.7028, 266.5666) -> (-214.8299, 280.248)
  spline S3 degree 5 poles (-213.7541, 291.5012) (-213.7836, 292.1337) (-213.9165, 293.5506) (-214.3357, 296.1342) (-215.3059, 300.4504) (-217.0551, 306.9808) (-219.1416, 314.1905) (-221.3444, 321.5493) (-223.447, 328.5165) (-225.2663, 334.6064) (-226.678, 339.4493) (-227.6481, 342.8655) (-228.2526, 344.9081) (-228.7265, 345.9852) (-229.415, 346.7173) (-230.5211, 347.2402) (-231.9417, 346.7519) (-233.4976, 344.3536) (-235.4615, 340.7393) (-237.9174, 336.5993) (-240.7362, 332.3678) (-243.6759, 328.3703) (-246.4235, 324.7873) (-248.6618, 321.698) (-250.1239, 319.0883) (-250.6571, 316.8737) (-250.2721, 314.9163) (-249.0801, 313.0601) (-247.2465, 311.16) (-244.9297, 309.119) (-242.2549, 306.9017) (-239.3271, 304.5172) (-236.2338, 302.0107) (-233.052, 299.4513) (-229.8531, 296.9221) (-226.7094, 294.5083) (-223.6983, 292.2901) (-220.9029, 290.3618) (-218.4131, 288.8445) (-216.3267, 287.9051) (-214.7483, 287.7655) (-213.986, 288.5405) (-213.7397, 289.7559) (-213.7247, 290.8688) (-213.7541, 291.5012) knots 0 0 0 0 0 0 0.025 0.05 0.075 0.1 0.125 0.15 0.175 0.2 0.225 0.25 0.275 0.3 0.325 0.35 0.375 0.4 0.425 0.45 0.475 0.5 0.525 0.55 0.575 0.6 0.625 0.65 0.675 0.7 0.725 0.75 0.775 0.8 0.825 0.85 0.875 0.9 0.925 0.95 0.975 1 1 1 1 1 1
  line L38 (-229, 351) -> (-237, 339)
  spline S4 degree 5 poles (-261, 320) (-260.7774, 319.9589) (-260.296, 319.9643) (-259.4625, 320.2428) (-258.1325, 321.1584) (-256.169, 323.121) (-254.0011, 325.7467) (-251.739, 328.8478) (-249.4883, 332.2331) (-247.3274, 335.7454) (-245.3055, 339.2672) (-243.4488, 342.7117) (-241.7644, 346.0192) (-240.2451, 349.1514) (-238.8737, 352.0857) (-237.6281, 354.8109) (-236.4846, 357.3206) (-235.4258, 359.6112) (-234.4564, 361.6897) (-233.6206, 363.5797) (-233.0136, 365.3267) (-232.8084, 367.0089) (-233.2246, 368.7247) (-234.4249, 370.5487) (-236.4437, 372.5039) (-239.0716, 374.5107) (-241.9507, 376.4378) (-244.6888, 378.1513) (-247.0272, 379.6106) (-248.853, 380.8435) (-250.59, 382.2095) (-252.6141, 383.9228) (-254.5082, 385.553) (-255.9404, 386.771) (-256.8623, 387.5494) (-258.3073, 388.9023) (-260.3731, 390.8134) (-262.725, 392.7952) (-264.822, 394.1558) (-266.2188, 394.3429) (-266.8921, 393.3204) (-267.1118, 391.4187) (-267.1481, 388.996) (-267.134, 386.2763) (-267.1221, 383.4019) (-267.1026, 380.4443) (-267.0374, 377.4316) (-266.8857, 374.368) (-266.6365, 371.2585) (-266.3041, 368.1107) (-265.9189, 364.9337) (-265.5197, 361.7382) (-265.1452, 358.5361) (-264.827, 355.3399) (-264.5793, 352.1629) (-264.3983, 349.0181) (-264.2687, 345.918) (-264.1682, 342.8735) (-264.0738, 339.8935) (-263.9654, 336.984) (-263.8335, 334.147) (-263.6787, 331.3832) (-263.501, 328.7082) (-263.2907, 326.1645) (-263.0185, 323.8353) (-262.6258, 321.8583) (-262.1382, 320.7217) (-261.6314, 320.2111) (-261.2226, 320.0411) (-261, 320) knots 0 0 0 0 0 0 0.01538462 0.03076923 0.04615385 0.06153846 0.07692308 0.09230769 0.10769231 0.12307692 0.13846154 0.15384615 0.16923077 0.18461538 0.2 0.21538462 0.23076923 0.24615385 0.26153846 0.27692308 0.29230769 0.30769231 0.32307692 0.33846154 0.35384615 0.36923077 0.38461538 0.4 0.41538462 0.43076923 0.44615385 0.46153846 0.47692308 0.49230769 0.50769231 0.52307692 0.53846154 0.55384615 0.56923077 0.58461538 0.6 0.61538462 0.63076923 0.64615385 0.66153846 0.67692308 0.69230769 0.70769231 0.72307692 0.73846154 0.75384615 0.76923077 0.78461538 0.8 0.81538462 0.83076923 0.84615385 0.86153846 0.87692308 0.89230769 0.90769231 0.92307692 0.93846154 0.95384615 0.96923077 0.98461538 1 1 1 1 1 1
  line L39 (-252.1641, 383.4813) -> (-260.6592, 390.8724)
  line L40 (-243.1248, 376.6611) -> (-254.8752, 385.339)
  spline S5 degree 5 poles (-231.7906, 374.6038) (-232.1085, 374.5208) (-232.851, 374.4896) (-234.2798, 374.8383) (-236.7582, 376.0277) (-240.548, 378.4434) (-244.694, 381.4466) (-248.8407, 384.6832) (-252.6635, 387.8353) (-255.9201, 390.6713) (-258.5019, 393.0953) (-260.4872, 395.1985) (-262.0644, 397.18) (-263.455, 399.2654) (-264.8371, 401.6282) (-266.2667, 404.3068) (-267.6058, 407.1298) (-268.6144, 409.8039) (-269.0428, 412) (-268.7121, 413.4336) (-267.6286, 413.9612) (-265.9511, 413.6215) (-263.7992, 412.6594) (-261.1969, 411.5005) (-258.172, 410.6183) (-254.8307, 410.4192) (-251.4272, 411.1358) (-248.4842, 412.6799) (-246.1926, 414.6246) (-244.5652, 416.391) (-243.4659, 417.3808) (-242.6867, 417.1356) (-242.0021, 415.4706) (-241.201, 412.4145) (-240.1185, 408.1637) (-238.6668, 403.0322) (-236.8701, 397.4028) (-234.8887, 391.6809) (-232.9697, 386.2702) (-231.4057, 381.5458) (-230.4896, 377.828) (-230.4758, 375.8505) (-230.9436, 374.9872) (-231.4727, 374.6867) (-231.7906, 374.6038) knots 0 0 0 0 0 0 0.025 0.05 0.075 0.1 0.125 0.15 0.175 0.2 0.225 0.25 0.275 0.3 0.325 0.35 0.375 0.4 0.425 0.45 0.475 0.5 0.525 0.55 0.575 0.6 0.625 0.65 0.675 0.7 0.725 0.75 0.775 0.8 0.825 0.85 0.875 0.9 0.925 0.95 0.975 1 1 1 1 1 1
  line L41 (-263.1838, 408.8802) -> (-243.4121, 412.833)
  spline S6 degree 5 poles (-213.9418, 208.154) (-214.0696, 208.5256) (-214.1797, 209.275) (-213.9048, 210.4054) (-212.7024, 211.8749) (-210.1263, 213.5214) (-206.9221, 214.8595) (-203.5777, 215.7898) (-200.5393, 216.2433) (-198.1353, 216.19) (-196.4747, 215.6545) (-195.4767, 214.7047) (-194.9497, 213.4312) (-194.6519, 211.9313) (-194.3624, 210.2884) (-193.9221, 208.5769) (-193.2802, 206.8702) (-192.5257, 205.2474) (-191.9595, 203.8037) (-192.0173, 202.6437) (-193.0886, 201.8616) (-195.339, 201.5236) (-198.6058, 201.6547) (-202.5179, 202.2474) (-206.5692, 203.2643) (-210.2085, 204.6435) (-212.3788, 205.9701) (-213.413, 207.0453) (-213.814, 207.7824) (-213.9418, 208.154) knots 0 0 0 0 0 0 0.04 0.08 0.12 0.16 0.2 0.24 0.28 0.32 0.36 0.4 0.44 0.48 0.52 0.56 0.6 0.64 0.68 0.72 0.76 0.8 0.84 0.88 0.92 0.96 1 1 1 1 1 1
  spline S7 degree 5 poles (-183, 198) (-182.8217, 198.0165) (-182.557, 198.2746) (-182.4163, 199.3066) (-182.5436, 201.685) (-182.4662, 205.1979) (-181.4757, 208.1349) (-179.2884, 209.7746) (-176.4408, 210.3) (-173.9796, 210.4944) (-172.9787, 211.2465) (-174.0981, 213.105) (-177.1726, 215.8633) (-181.5132, 218.8579) (-186.1365, 221.1984) (-190.0241, 222.0271) (-192.3467, 220.7457) (-192.7517, 217.3103) (-191.4825, 212.3413) (-189.1238, 206.8171) (-186.4319, 201.8613) (-184.5946, 199.1691) (-183.6268, 198.1755) (-183.1783, 197.9835) (-183, 198) knots 0 0 0 0 0 0 0.05 0.1 0.15 0.2 0.25 0.3 0.35 0.4 0.45 0.5 0.55 0.6 0.65 0.7 0.75 0.8 0.85 0.9 0.95 1 1 1 1 1 1
  point P0 (-216.7663, 273.4073)
  point P1 (-218.653, 278.8454)
  point P2 (-247.5082, 299.4879)
  point P3 (-252.8353, 297.0464)
  point P4 (-251.9475, 270.8547)
  point P5 (-248.0631, 263.7519)
  point P6 (-235.6269, 260.2006)
  point P7 (-228, 344)
  point P8 (-229.5217, 346.6604)
  point P9 (-233, 345)
  point P10 (-249.7631, 319.49)
  point P11 (-248, 312)
  point P12 (-230.5037, 297.4482)
  point P13 (-216, 288)
  point P14 (-251, 330)
  point P15 (-238, 354)
  point P16 (-233.3456, 364.4742)
  point P17 (-235, 371)
  point P18 (-249, 381)
  point P19 (-256.4117, 387.1769)
  point P20 (-265, 394)
  point P21 (-267, 392)
  point P22 (-267, 377)
  point P23 (-265, 357)
  point P24 (-264, 338)
  point P25 (-263, 324)
  point P26 (-255.7906, 390.6038)
  point P27 (-264.7906, 401.6038)
  point P28 (-268.7997, 412.5359)
  point P29 (-266.4959, 413.6529)
  point P30 (-253.298, 410.8566)
  point P31 (-243.6324, 417.0388)
  point P32 (-238.7906, 403.6038)
  point P33 (-199.9418, 216.154)
  point P34 (-194.9418, 213.154)
  point P35 (-192.9418, 206.154)
  point P36 (-192.9418, 202.154)
  point P37 (-180.825, 208.2725)
  point P38 (-173.5028, 211.4008)
  point P39 (-191.3442, 220.8543)
  dimension "d252" = 1
  dimension "d253" = 1
  constraint tangent S0 A7
  constraint tangent L5 A7
  constraint tangent S0 A8
  constraint tangent L5 A8
  constraint coincident L9.start L34.end
  constraint midpoint P6 L35
  constraint midpoint S2.start L36
  constraint midpoint P0 L37
  constraint midpoint P9 L38
  constraint midpoint P19 L39
  constraint midpoint P18 L40
  constraint midpoint P30 L41
  measures "d252" radius of A7
  measures "d253" radius of A8
extrude "Extrude1'''" cut sketch "Sketch13" against normal through all contours S0 L5 A7 A8 | S1 | S2 L35 | S2 L35 | S2 L35 | S3 | S4 | S5 | S6 | S7 bodies 7 in component "Brazo_superior"
ref_plane "WorkPlane6" through (-80, 0, 0) normal (1, 0, 0) x (0, 1, 0)
mirror "Mirror1" about plane through (-80, 0, 0) normal (1, 0, 0) of bodies 4 makes body 17 in component "Brazo_inferior"
extrude "Extrude5'" add 1 faces at (-85, -221.2604, 251.0133) along direction (1, 0, 0) up to surface (10 mm away) on bodies 4 bodies 4 17 in component "Brazo_inferior"
sketch "Sketch1 (2)" plane through (-80, 0, 0) normal (1, 0, 0) x (0, 1, 0) in component "Brazo_inferior"
  line L0 (-79.9597, 105.9784) -> (-121.9147, 90.708)
  arc A0 (-121.9147, 90.708) -> (-31.2551, 19.9998) centre (380.3227, 641.1856) ccw
  line L1 (-31.2551, 19.9998) -> (-23.7809, 62.3878)
  arc A1 (-79.9597, 105.9784) -> (-23.7809, 62.3878) centre (380.3227, 641.1856) ccw
  arc A2 (-168.2204, 196.8803) -> (-84.2819, 109.7261) centre (380.3227, 641.1856) ccw
  line L2 (-168.2204, 196.8803) -> (-177.0785, 146.6434)
  arc A3 (-177.0785, 146.6434) -> (-126.061, 94.5198) centre (380.3227, 641.1856) ccw
  line L3 (-126.061, 94.5198) -> (-84.2819, 109.7261)
  arc A4 (-19.2562, 59.2549) -> (53.7571, 15.3569) centre (380.3227, 641.1856) ccw
  line L4 (-19.2562, 59.2549) -> (-26.7053, 17.0091)
  arc A5 (-26.7053, 17.0091) -> (4.8259, -2.4526) centre (380.3227, 641.1856) ccw
  line L5 (4.8259, -2.4526) -> (53.7571, 15.3569)
  arc A6 (-203.1179, 177.6501) -> (-181.3078, 151.4518) centre (380.3227, 641.1856) ccw
  line L6 (-181.3078, 151.4518) -> (-172.3826, 202.0689)
  arc A7 (-172.3826, 202.0689) -> (-203.1179, 177.6501) centre (-187.7502, 189.8595) ccw
  arc A8 (41.2897, -22.384) -> (59.7882, 12.2312) centre (50.2197, -4.9058) ccw
  line L7 (59.7882, 12.2312) -> (10.4773, -5.7166)
  arc A9 (10.4773, -5.7166) -> (41.2897, -22.384) centre (380.3227, 641.1856) ccw
  circle A10 centre (-223.3374, 249.0861) radius 8.5
  line L8 (-249.6006, 234.5968) -> (-241.9437, 238.8211)
  arc A11 (-241.9437, 238.8211) -> (-240.9623, 242.2177) centre (-243.1513, 241.0101) ccw
  line L9 (-240.9623, 242.2177) -> (-248.2082, 255.3516)
  arc A12 (-247.2269, 258.7482) -> (-248.2082, 255.3516) centre (-246.0193, 256.5592) ccw
  line L10 (-247.2269, 258.7482) -> (-218.7703, 274.4476)
  arc A13 (-215.3737, 273.4663) -> (-218.7703, 274.4476) centre (-217.5627, 272.2586) ccw
  line L11 (-215.3737, 273.4663) -> (-208.1278, 260.3325)
  arc A14 (-208.1278, 260.3325) -> (-204.7312, 259.3511) centre (-205.9388, 261.5401) ccw
  line L12 (-204.7312, 259.3511) -> (-179.3789, 273.3379)
  arc A15 (-175.9823, 272.3566) -> (-179.3789, 273.3379) centre (-178.1713, 271.1489) ccw
  line L13 (-175.9823, 272.3566) -> (-171.1517, 263.6007)
  arc A16 (-172.133, 260.2041) -> (-171.1517, 263.6007) centre (-173.3407, 262.3931) ccw
  line L14 (-172.133, 260.2041) -> (-185.201, 252.9945)
  arc A17 (-185.201, 252.9945) -> (-186.1426, 249.5286) centre (-183.9934, 250.8056) ccw
  arc A18 (-186.1426, 249.5286) -> (95.8875, 14.6255) centre (286.6925, 530.468) ccw
  arc A19 (95.8875, 14.6255) -> (99.1261, 16.1784) centre (96.7548, 16.9703) ccw
  line L15 (99.1261, 16.1784) -> (103.7889, 30.1406)
  arc A20 (106.9521, 31.72) -> (103.7889, 30.1406) centre (106.1602, 29.3487) ccw
  line L16 (106.9521, 31.72) -> (116.4371, 28.5523)
  arc A21 (118.0165, 25.3892) -> (116.4371, 28.5523) centre (115.6452, 26.1811) ccw
  line L17 (118.0165, 25.3892) -> (92.6771, -50.4864)
  arc A22 (89.5042, -52.0625) -> (92.6771, -50.4864) centre (90.3058, -49.6945) ccw
  arc A23 (-250.577, 231.1913) -> (89.5042, -52.0625) centre (286.6925, 530.468) ccw
  arc A24 (-249.6006, 234.5968) -> (-250.577, 231.1913) centre (-248.3929, 232.4079) ccw
  circle A25 centre (85.5661, -40.2098) radius 6
  circle A26 centre (99.8204, 2.4729) radius 6
  circle A27 centre (-20.3718, 67.3252) radius 5
  circle A28 centre (-30.1147, 12.0701) radius 5
  circle A29 centre (-171.8436, 133.1719) radius 5
  circle A30 centre (-145.8264, 183.2611) radius 5
  line L18 (96.7376, -38.3276) -> (67.5802, -28.5902) construction
  line L19 (85.5661, -40.2098) -> (105.2632, 18.7705) construction
  line L20 (-26.7053, 17.0091) -> (-31.2551, 19.9998) construction
  line L21 (-30.6641, 8.9544) -> (-17.5305, 83.4385) construction
  line L22 (-19.2562, 59.2549) -> (-23.7809, 62.3878) construction
  dimension "d260" = 12
  dimension "d261" = 12
  dimension "d262" = 10
  dimension "d263" = 10
  dimension "d264" = 10
  dimension "d265" = 10
  dimension "d266" = 10
  dimension "d267" = 30
  dimension "d268" = 45
  dimension "d269" = 6
  dimension "d270" = 6
  constraint coincident L17 L18.start
  constraint perpendicular L17 L18
  constraint coincident A25.centre L19.start
  constraint perpendicular L18 L19
  constraint coincident A26.centre L19
  constraint coincident L4.end A5.start
  constraint coincident A0.end L1.start
  constraint parallel L1 L21
  constraint coincident A27.centre L21
  constraint coincident A28.centre L21
  constraint coincident A4.start L4.start
  constraint coincident L1.end A1.end
  measures "d260" diameter of A25
  measures "d261" diameter of A26
  measures "d262" diameter of A27
  measures "d263" diameter of A28
  measures "d264" diameter of A29
  measures "d265" diameter of A30
  measures "d266" distance of L17 A25.centre
  measures "d267" distance of L16 A26.centre
  measures "d268" distance of A25.centre A26.centre
  measures "d269" distance of A27.centre L22
  measures "d270" distance of A28.centre L20
extrude "Extrude6'" add sketch "Sketch1 (2)" along normal mid plane 160 contours A25 | A26 | A27 | A28 bodies 4 in component "Brazo_inferior"
mirror "Mirror1'" about plane through (-80, 0, 0) normal (1, 0, 0) of bodies 7 makes body 18 in component "Brazo_superior"
extrude "Extrude2''" add 1 faces at (-70, -172.9633, 203.6964) along direction (-1, 0, 0) up to surface (20 mm away) on bodies 7 bodies 7 18 in component "Brazo_superior"